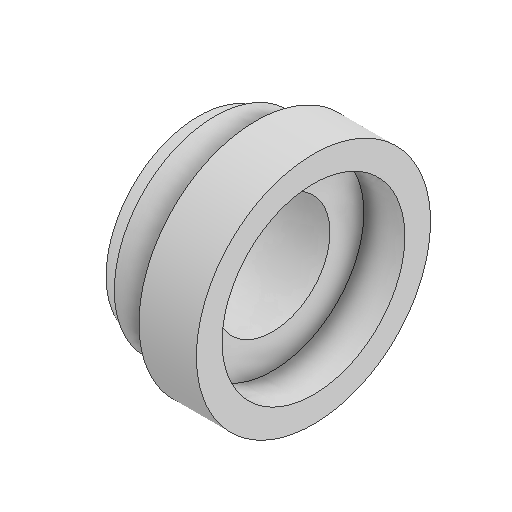
# Autodesk Inventor part: am3298_bearing_adapter
Saved by Autodesk Inventor 2025 (Build 290162000, 162)
## iProperties
Created: 2024-06-25
Part Number: am3298_bearing_adapter
Material: Generic
Document SubType Name: Modeling
Designer: derm
Density: 1 g/cm^3
Appearance: Default
Author: derm
Autodesk Inventor part; units mm, degrees
ref_plane "YZ Plane" through (0, 0, 0) normal (1, 0, 0) x (0, 1, 0)
ref_plane "XZ Plane" through (0, 0, 0) normal (0, 1, 0) x (-1, 0, 0)
ref_plane "XY Plane" through (0, 0, 0) normal (0, 0, 1) x (1, 0, 0)
sketch "Sketch1" plane through (0, 0, 0) normal (1, 0, 0) x (0, 1, 0)
  circle A0 centre (0, 0) radius 11.125
  circle A1 centre (0, 0) radius 14.25
  dimension "d0" = 22.25
  dimension "d1" = 28.5
  constraints: 2 centre point, 2 coincident
  measures "d0" diameter of A0
  measures "d1" diameter of A1
extrude "Extrusion1" add sketch "Sketch1" against normal blind 7
sketch "Sketch2" plane through (-7, 0, 0) normal (-1, 0, 0) x (0, 0, 1)
  circle A0 centre (0, 0) radius 14.25 projected
  circle A1 centre (0, 0) radius 11.125 projected
  circle A2 centre (0, 0) radius 12.25
  circle A3 centre (0, 0) radius 14.25 projected
  circle A4 centre (0, 0) radius 7
  dimension "d4" = 24.5
  dimension "d5" = 14
  constraints: 2 centre point, 2 coincident
  measures "d4" diameter of A2
  measures "d5" diameter of A4
extrude "Extrusion2" add sketch "Sketch2" along normal blind 7 contours A1 | A2
sketch "Sketch3" plane through (-7, 0, 0) normal (1, 0, 0) x (0, 0, -1)
  circle A0 centre (0, 0) radius 7 projected
  circle A1 centre (0, 0) radius 11.125 projected
extrude "Extrusion3" add sketch "Sketch3" along normal blind 2
chamfer "Chamfer1" distance 1 distance2 2 1 edges at (-14, 0, -12.25) measured on face at (-14, -0.9772, 10.3813)
body "Solid1"
